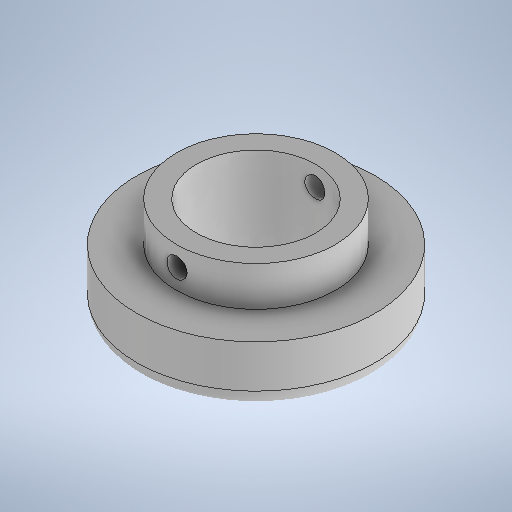
# Autodesk Inventor part: 03
Saved by Autodesk Inventor 2025.1 (Build 291241000, 241)
## iProperties
Created: 2024-09-12
Part Number: 03
Material: Generisch
Document SubType Name: Modeling
Designer: ffogue
Density: 1 g/cm^3
Appearance: Vorgabe
Author: ffogue
Autodesk Inventor part; units mm, degrees
ref_plane "YZ Plane" through (0, 0, 0) normal (1, 0, 0) x (0, 1, 0)
ref_plane "XY Plane" through (0, 0, 0) normal (0, 0, 1) x (1, 0, 0)
sketch "Sketch1" plane through (0, 0, 0) normal (1, 0, 0) x (0, 1, 0)
  line L0 (0, 0) -> (4, 0)
  line L1 (4, 0) -> (4, -2)
  line L2 (4, -2) -> (6, -2)
  line L3 (6, -2) -> (6, -5)
  line L4 (6, -5) -> (0, -5)
  line L5 (0, -5) -> (0, 0)
  point P0 (3, -5)
  dimension "d0" = 5
  dimension "d1" = 2
  dimension "d2" = 8
  dimension "d3" = 12
  constraints: 12 end point, 5 perpendicular, 1 horizontal, 1 midpoint
  measures "d0" distance from line of point (3, -5) L0
  measures "d1" distance of L0.end L1.end
  measures "d2" diameter of L1 L5
  measures "d3" diameter of L3 L5
revolve "Revolution1" add sketch "Sketch1" angle 360 about axis through (0, 0, -5) along (0, 0, 1)
sketch "Sketch2" plane through (0, 0, 0) normal (0, 0, 1) x (1, 0, 0)
  circle A0 centre (0, 0) radius 4 projected
  constraints: 1 coincident
hole "Hole1" at (0, 0, 0) direction (0, 0, -1) diameter 6 depth 5
fillet "Fillet1" radius 0.85 1 edges at (0, -6, -5)
ref_plane "Work Plane1" through (0, 4, 0) normal (0, 1, 0) x (-1, 0, 0)
sketch "Sketch3" plane through (0, 4, 0) normal (0, 1, 0) x (-1, 0, 0)
  point P0 (0, 0)
  point P1 (0, -1)
  dimension "d14" = 1
  constraints: 1 vertical alignment
  measures "d14" distance of point (0, 0) point (0, -1)
hole "Hole2" at (0, 4, -1) direction (0, -1, 0) diameter 1 end through all
body "Solid1"
